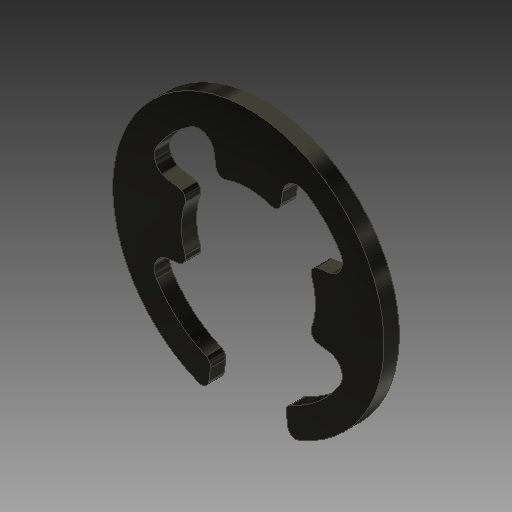
# Autodesk Inventor part: External Klipring for 500 shaft (am-0206)
Saved by Autodesk Inventor 2018 (Build 220112000, 112)
## iProperties
Created: 2015-02-08
Part Number: External Klipring for 500 shaft (am-0206)
Material: Steel, Carbon
Document SubType Name: Modeling
Designer: TODD D MILLER
Mass: 1.93755 g
Surface Area: 5.50007 cm^2
Volume: 0.246822 cm^3
Density: 7.85 g/cm^3
Appearance: Gunmetal
Description: External Klipring for 500 shaft
Vendor: AndyMark
Stock Number: am-0206
Author: TODD D MILLER
Autodesk Inventor part; units mm, degrees
ref_plane "YZ Plane" through (0, 0, 0) normal (1, 0, 0) x (0, 1, 0)
ref_plane "XZ Plane" through (0, 0, 0) normal (0, 1, 0) x (-1, 0, 0)
ref_plane "XY Plane" through (0, 0, 0) normal (0, 0, 1) x (1, 0, 0)
sketch "Sketch1" plane through (0, 0, 0) normal (0, 0, 1) x (1, 0, 0)
  circle A0 centre (0, 0) radius 5.588
  circle A1 centre (0, 0) radius 11.303
  dimension "d0" = 11.176
  dimension "d1" = 22.606
  constraints: 2 centre point, 2 coincident
  measures "d0" diameter of A0
  measures "d1" diameter of A1
extrude "Extrusion1" add sketch "Sketch1" along normal mid plane 1.27
sketch "Sketch2" plane through (0, 0, 0.635) normal (0, 0, 1) x (1, 0, 0)
  circle A0 centre (0, 0) radius 11.303 projected
  circle A1 centre (0, 0) radius 9.017
  line L0 (0, 0) -> (-7.9924, 7.9924) construction
  line L1 (0, 0) -> (-16.0053, 0) construction
  line L2 (-3.0848, 8.4729) -> (-2.2451, 2.2451)
  line L3 (-2.2451, 2.2451) -> (-8.4729, 3.0848)
  dimension "d4" = 2.286
  dimension "d5" = 45
  dimension "d6" = 3.175
  dimension "d7" = 7.62
  constraints: 8 end point, 2 point on circle, 1 centre point, 1 horizontal, 1 point on line, 3 other
  measures "d5" angle of L1 L0
  measures "d6" distance of L0.start L2.end
  measures "d7" distance of L2.start L3.end
extrude "Extrusion2" cut sketch "Sketch2" against normal through all contours L2 L3 A1 picked at (-6.1075, 3.3917)
pattern_circular "Circular Pattern1" count 4 over 360 about axis through (0, 0, -10) along (0, 0, 1) of "Extrusion2"
sketch "Sketch3" plane through (0, 0, 0.635) normal (0, 0, 1) x (1, 0, 0)
  line L0 (2.6087, 4.9417) -> (3.0848, 8.4729) projected
  arc A0 (8.4729, 3.0848) -> (3.0848, 8.4729) centre (0, 0) ccw projected
  line L1 (8.4729, 3.0848) -> (4.9417, 2.6087) projected
  arc A1 (4.9417, -2.6087) -> (4.9417, 2.6087) centre (0, 0) ccw projected
  line L2 (4.9417, -2.6087) -> (8.4729, -3.0848) projected
  arc A2 (3.0848, -8.4729) -> (8.4729, -3.0848) centre (0, 0) ccw projected
  line L3 (3.0848, -8.4729) -> (2.6087, -4.9417) projected
  arc A3 (-2.6087, -4.9417) -> (2.6087, -4.9417) centre (0, 0) ccw projected
  line L4 (-2.6087, -4.9417) -> (-3.0848, -8.4729) projected
  arc A4 (-8.4729, -3.0848) -> (-3.0848, -8.4729) centre (0, 0) ccw projected
  line L5 (-8.4729, -3.0848) -> (-4.9417, -2.6087) projected
  arc A5 (-4.9417, 2.6087) -> (-4.9417, -2.6087) centre (0, 0) ccw projected
  line L6 (-4.9417, 2.6087) -> (-8.4729, 3.0848) projected
  arc A6 (-3.0848, 8.4729) -> (-8.4729, 3.0848) centre (0, 0) ccw projected
  line L7 (-3.0848, 8.4729) -> (-2.6087, 4.9417) projected
  arc A7 (2.6087, 4.9417) -> (-2.6087, 4.9417) centre (0, 0) ccw projected
  circle A8 centre (0, 0) radius 11.303 projected
  line L8 (-3.0848, -8.4729) -> (-3.3959, -10.7808)
  circle A9 centre (0, 0) radius 11.303 projected
  line L9 (3.0848, -8.4729) -> (3.3959, -10.7808)
  line L10 (-2.6087, -4.9417) -> (-3.0848, -8.4729) projected
  line L11 (3.0848, -8.4729) -> (2.6087, -4.9417) projected
  constraints: 4 end point, 4 point on circle, 2 collinear
extrude "Extrusion3" cut sketch "Sketch3" against normal through all contours L9 A8 L8 L4 A3 L3
fillet "Fillet1" radius 1.27 6 edges at (-8.4729, -3.0848, 0) (8.4729, -3.0848, 0) (8.4729, 3.0848, 0) (3.0848, 8.4729, 0) (-3.0848, 8.4729, 0) (-8.4729, 3.0848, 0)
fillet "Fillet1" radius 0.635 10 edges at (-4.9417, -2.6087, 0) (-4.9417, 2.6087, 0) (-2.6087, 4.9417, 0) (2.6087, 4.9417, 0) (4.9417, 2.6087, 0) (4.9417, -2.6087, 0) (-3.0848, -8.4729, 0) (-3.3959, -10.7808, 0) (3.3959, -10.7808, 0) (3.0848, -8.4729, 0)
body "Solid1"
